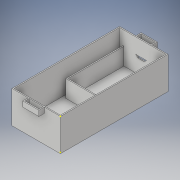
# Autodesk Inventor part: Pièce1
Saved by Autodesk Inventor 2017 (Build 210142000, 142)
## iProperties
Created: 2020-03-28
Part Number: Pièce1
Material: Generic
Document SubType Name: Modeling
Designer: LUC
Density: 1 g/cm^3
Appearance: Default
Author: LUC
Autodesk Inventor part; units mm, degrees
ref_plane "YZ Plane" through (0, 0, 0) normal (1, 0, 0) x (0, 1, 0)
ref_plane "XZ Plane" through (0, 0, 0) normal (0, 1, 0) x (-1, 0, 0)
ref_plane "XY Plane" through (0, 0, 0) normal (0, 0, 1) x (1, 0, 0)
sketch "Esquisse1" plane through (0, 0, 0) normal (0, 1, 0) x (-1, 0, 0)
  line L0 (0, 0) -> (0, -100)
  line L1 (0, -100) -> (45, -100)
  line L2 (45, -100) -> (45, 0)
  line L3 (45, 0) -> (0, 0)
  dimension "d1" = 100
  dimension "d2" = 45
  constraints: 8 end point, 3 perpendicular, 1 vertical
  measures "d1" distance of L0.start L0.end
  measures "d2" distance of L0.end L1.end
extrude "Extrusion1" add sketch "Esquisse1" along normal blind 30
shell "Coque1" thickness 1 removed faces 1 at (-15, 30, -66.6667)
sketch "Esquisse2" plane through (-44, 1, -99) normal (0, 1, 0) x (1, 0, 0)
  point P0 (44, -99)
sketch "Esquisse3" plane through (-44, 1, -99) normal (0, 1, 0) x (1, 0, 0)
  point P0 (44, -99)
sketch "Esquisse4" plane through (-44, 1, -99) normal (0, 1, 0) x (1, 0, 0)
  line L0 (43, 0) -> (0, 0) projected
  line L1 (0, 0) -> (3, 0)
  line L2 (3, 0) -> (3, -53)
  line L3 (3, -53) -> (40, -53)
  line L4 (44, -99) -> (44, 1) projected
  line L5 (40, -53) -> (40, 0)
  line L6 (40, 0) -> (3, 0)
  line L7 (44, 1) -> (-1, 1) projected
  dimension "d6" = 3
  dimension "d7" = 53
  dimension "d8" = 37
  constraints: 10 end point, 3 perpendicular, 2 point on line, 1 parallel
  measures "d6" distance of L0.end L1.end
  measures "d7" distance of L1.end L2.end
  measures "d8" distance of L2.end L3.end
extrude "Extrusion2" add sketch "Esquisse4" along normal blind 16
sketch "Esquisse5" plane through (0, 0, -100) normal (0, 0, -1) x (-1, 0, 0)
  line L0 (45, 0) -> (45, 14)
  line L1 (45, 0) -> (45, 30) projected
  line L2 (19.011, 16) -> (29.011, 16)
  line L3 (19.011, 16) -> (27.012, 16)
  line L4 (19.011, 16) -> (21.011, 14)
  line L5 (29.011, 16) -> (33, 16)
  line L6 (29.011, 16) -> (27.011, 14)
  line L7 (21.011, 14) -> (27.011, 14)
  point P0 (0, 0)
  dimension "d17" = 10
  dimension "d18" = 8.001
  constraints: 14 end point, 3 point on line, 1 horizontal
  measures "d17" distance of L2.start L2.end
  measures "d18" distance of L2.start L3.end
shell "Coque2" thickness 1 removed faces 1 at (-28.6667, 17, -81.3333)
extrude "Extrusion4" cut sketch "Esquisse5" against normal blind 10
sketch "Esquisse7" plane through (-45, 0, 0) normal (0, 0, 1) x (1, 0, 0)
  line L0 (0, 30) -> (45, 30) projected
  line L1 (15.069, 30) -> (30.069, 30)
  line L2 (15.069, 30) -> (30.069, 30)
  line L3 (30.069, 30) -> (30.069, 24.9829)
  line L4 (30.069, 24.9829) -> (15.069, 24.9829)
  line L5 (15.069, 24.9829) -> (15.069, 30)
  line L6 (15.069, 30) -> (30.069, 30)
  line L7 (30.069, 24.9829) -> (15.069, 24.9829)
  line L8 (0, 0) -> (45, 0) projected
  line L9 (45, 0) -> (45, 30) projected
  line L10 (0, 30) -> (45, 30) projected
  line L11 (0, 0) -> (0, 30) projected
  dimension "d24" = 15
  constraints: 14 end point, 3 equal length, 2 horizontal, 2 point on line, 1 perpendicular
  measures "d24" distance of L1.start L1.end
extrude "Extrusion5" add sketch "Esquisse7" along normal blind 5 contours L0 L3 L4 L5
sketch "Esquisse11" plane through (0, 30, 0) normal (0, 1, 0) x (1, 0, 0)
  point P0 (0, 0)
shell "Coque3" thickness 1 removed faces 1 at (-0.3333, 30, -33.6667)
sketch "Esquisse12" plane through (0, 0, -100) normal (0, 0, -1) x (-1, 0, 0)
  line L0 (14.931, 30) -> (0, 30) projected
  line L1 (14.931, 30) -> (29.931, 30)
  line L2 (44, 30) -> (1, 30) projected
  line L3 (29.931, 24.9829) -> (29.931, 30) projected
  line L4 (14.931, 30) -> (29.931, 30)
  line L5 (29.931, 30) -> (29.931, 25)
  line L6 (29.931, 25) -> (14.931, 25)
  line L7 (14.931, 25) -> (14.931, 30)
  point P0 (0, 0)
  dimension "d30" = 15
  dimension "d31" = 5
  constraints: 10 end point, 2 parallel, 2 point on line, 1 horizontal, 1 perpendicular
  measures "d30" distance of L0.start L1.end
  measures "d31" distance of L4.end L5.end
extrude "Extrusion6" add sketch "Esquisse12" along normal blind 5
shell "Coque4" thickness 1 removed faces 1 at (-44.6667, 30, -33.6667)
